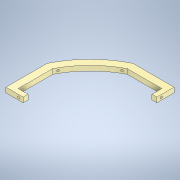
# Autodesk Inventor part: insert_8in
Saved by Autodesk Inventor 2021 (Build 250183000, 183)
## iProperties
Created: 2020-10-07
Part Number: insert_8in
Material: Generic
Document SubType Name: Modeling
Designer: dsouthall
Density: 1 g/cm^3
Appearance: Default
Author: dsouthall
Autodesk Inventor part; units mm, degrees
ref_plane "YZ Plane" through (0, 0, 0) normal (1, 0, 0) x (0, 1, 0)
ref_plane "XY Plane" through (0, 0, 0) normal (0, 0, 1) x (1, 0, 0)
sketch "Sketch1" plane through (0, 0, 0) normal (0, 1, 0) x (-1, 0, 0)
  line L0 (226.205, -0.8) -> (-105.3043, -0.8) construction
  line L1 (226.205, 0) -> (0, 0) construction
  line L2 (0, 0) -> (0, -248.1018) construction
  line L3 (0.8, -248.1018) -> (0.8, 57.2198) construction
  line L4 (226.205, -5.88) -> (-105.3043, -5.88) construction
  line L5 (5.88, -248.1018) -> (5.88, 57.2198) construction
  line L6 (69.985, -0.8) -> (87.765, -0.8)
  line L7 (87.765, -0.8) -> (87.765, -43.4351)
  line L8 (80.145, -5.88) -> (80.145, -41.6146)
  line L9 (69.985, -0.8) -> (69.985, -5.88)
  line L10 (69.985, -5.88) -> (80.145, -5.88)
  line L11 (0.8, -87.765) -> (43.4351, -87.765)
  line L12 (5.88, -80.145) -> (41.6146, -80.145)
  arc A0 (41.6146, -80.145) -> (80.145, -41.6146) centre (0, 0) ccw
  arc A1 (43.4351, -87.765) -> (87.765, -43.4351) centre (0, 0) ccw
  line L13 (0.8, -87.765) -> (0.8, -69.985)
  line L14 (0.8, -69.985) -> (5.88, -69.985)
  line L15 (5.88, -69.985) -> (5.88, -80.145)
  arc A2 (87.765, -43.4351) -> (97.925, 0) centre (0, 0) ccw construction
  line L16 (74.425, -0.8) -> (74.425, -5.88) construction
  line L17 (0, 0) -> (93.3789, -93.3789) construction
  line L18 (0, 0) -> (133.2097, -76.9087) construction
  line L19 (0, 0) -> (80.0181, -138.5954) construction
  point P0 (84.8055, -48.9625)
  point P1 (48.9625, -84.8055)
  dimension "d5" = 0.8
  dimension "d6" = 0.8
  dimension "d7" = 90
  dimension "d8" = 5.08
  dimension "d9" = 5.08
  dimension "d13" = 90
  dimension "d14" = 87.765
  dimension "d15" = 7.62
  dimension "d16" = 69.985
  dimension "d17" = 90
  dimension "d19" = 7.62
  dimension "d20" = 69.985
  dimension "d21" = 17.78
  dimension "d22" = 97.925
  dimension "d23" = 90.305
  dimension "d24" = 23.5
  dimension "d46" = 45
  dimension "d56" = 30
  dimension "d57" = 60
  constraints: 40 end point, 13 point on line, 8 point on circle, 5 parallel, 3 centre point, 3 coincident, 2 horizontal, 2 perpendicular, 1 collinear, 1 vertical
  measures "d5" distance between parallel lines of L1 L0
  measures "d6" distance between parallel lines of L2 L3
  measures "d7" angle of L2 L1
  measures "d8" distance between parallel lines of L0 L4
  measures "d9" distance between parallel lines of L3 L5
  measures "d13" angle of L0 L7
  measures "d14" horizontal distance of point (0, 0) L6.end
  measures "d15" distance between parallel lines of L7 L8
  measures "d16" horizontal distance of point (0, 0) L6.start
  measures "d17" angle of L3 L11
  measures "d19" distance between parallel lines of L12 L11
  measures "d20" distance from line of point (0, 0) L14
  measures "d21" distance of L11.start L13.end
  measures "d22" radius of A1
  measures "d23" radius of A0
  measures "d24" horizontal distance of L16.start A2.end
  measures "d46" angle of L17 L1
  measures "d56" angle of L18 L1
  measures "d57" angle of L19 L1
extrude "Extrusion1" add sketch "Sketch1" along normal blind 5.08
ref_plane "radial plane for hole1" through (0, 0, 0) normal (0, 0, 1) x (1, 0, 0)
sketch "sketch hole 1" plane through (0, 0, 0) normal (0, 0, 1) x (1, 0, 0)
  line L0 (-74.425, 0) -> (-74.425, 5.08) construction
  line L1 (-87.765, 5.08) -> (-69.985, 5.08) projected
  point P0 (0, 0)
  point P1 (-74.425, 2.54)
  dimension "d28" = 74.425
  dimension "d29" = 2.54
  constraints: 2 end point, 1 midpoint, 1 vertical
  measures "d28" distance from line of point (0, 0) L0
  measures "d29" distance from line of L1 point (-74.425, 2.54)
ref_plane "radial plane for hole2" through (0, 0, 0) normal (1, 0, 0) x (0, 0, -1)
hole "Hole2" at (0, 2.54, -74.425) direction (-1, 0, 0) diameter 2.4384 depth 12.2936 tip angle 118 clearance for "Flat Head Machine Screw (82)" size "#2" standard "Ansi Unified Screw Threads"
sketch "sketch hole 2" plane through (0, 0, 0) normal (1, 0, 0) x (0, 0, -1)
  line L0 (74.425, 5.3744) -> (74.425, -0.2944) construction
  line L1 (69.985, 5.08) -> (87.765, 5.08) construction
  point P0 (0, 0)
  point P1 (74.425, 2.54)
  dimension "d30" = 74.425
  dimension "d31" = 2.54
  constraints: 2 end point, 1 midpoint, 1 vertical
  measures "d30" distance from line of point (0, 0) L0
  measures "d31" distance from line of L1 point (74.425, 2.54)
hole "Hole1" at (-74.425, 2.54, 0) direction (0, 0, -1) diameter 2.4384 depth 12.2936 tip angle 118 clearance for "Flat Head Machine Screw (82)" size "#2" standard "Ansi Unified Screw Threads"
ref_plane "tangential plane for hole3" through (-69.2434, 0, -69.2434) normal (-0.7071068, 0, -0.7071068) x (0, -1, 0)
ref_plane "tangential plane for hole 4" through (-84.8055, 0, -48.9625) normal (-0.8660254, 0, -0.5) x (0, -1, 0)
ref_plane "tangential plane for hole 5" through (-48.9625, 0, -84.8055) normal (-0.5, 0, -0.8660254) x (0, -1, 0)
sketch "sketch hole 4" plane through (-84.8055, 0, -48.9625) normal (-0.8660254, 0, -0.5) x (0, -1, 0)
  line L0 (-5.08, 6.2666) -> (-5.08, -54.2892) projected
  line L1 (0, 6.2666) -> (0, -54.2892) projected
  point P0 (0, 0)
  point P1 (-2.54, 0)
  dimension "d58" = 5.08
  dimension "d59" = 2.54
  dimension "d60" = 0
  measures "d58" distance between parallel lines of L0 L1
  measures "d59" distance from line of L1 point (-2.54, 0)
  measures "d60" vertical distance of point (-2.54, 0) point (0, 0)
sketch "Sketch8" plane through (-48.9625, 0, -84.8055) normal (-0.5, 0, -0.8660254) x (0, -1, 0)
  line L0 (0, 54.2892) -> (0, -6.2666) projected
  line L1 (-5.08, 54.2892) -> (-5.08, -6.2666) projected
  point P0 (0, 0)
  point P1 (-2.54, 0)
  dimension "d61" = 5.08
  dimension "d62" = 2.54
  dimension "d63" = 0
  measures "d61" distance between parallel lines of L0 L1
  measures "d62" distance from line of L0 point (-2.54, 0)
  measures "d63" vertical distance of point (0, 0) point (-2.54, 0)
hole "Hole4" at (-84.8055, 2.54, -48.9625) direction (0.8660254, 0, 0.5) diameter 2.1565 depth 8.8646 tip angle 118 thread size "4-40 UNC" class "2B" standard "ANSI Unified Screw Threads"
hole "Hole5" at (-48.9625, 2.54, -84.8055) direction (0.5, 0, 0.8660254) diameter 2.1565 depth 8.8646 tip angle 118 thread size "4-40 UNC" class "2B" standard "ANSI Unified Screw Threads"
ref_plane "Work Plane8" through (0, 2.54, 0) normal (0, 1, 0) x (-1, 0, 0)
split "Split1" [suppressed]
equation "\"d6\" = d5"
equation "\"d9\" = d8"
equation "\"d17\" = d13"
equation "\"d19\" = d15"
equation "\"d20\" = d16"
equation "\"d21\" = d14 - d16"
equation "\"d46\" = 0.5 * d7"
equation "\"d56\" = 0.333333 * d7"
equation "\"d57\" = 0.666667 * d7"
equation "\"d28\" = d22 - d24"
equation "\"d30\" = d28"
equation "\"d59\" = 0.5 * d58"
equation "\"d62\" = 0.5 * d61"
body "Solid1"
